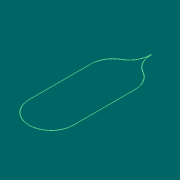
# Autodesk Inventor part: Fiber Loop
Saved by Autodesk Inventor 2016 (Build 200138000, 138)
## iProperties
Created: 2015-08-17
Part Number: Fiber Loop
Material: Glass
Document SubType Name: Modeling
Designer: Cosmic
Density: 2.18 g/cm^3
Appearance: Clear - Green 1
Author: Cosmic
Autodesk Inventor part; units mm, degrees
ref_plane "YZ Plane" through (0, 0, 0) normal (1, 0, 0) x (0, 1, 0)
ref_plane "XZ Plane" through (0, 0, 0) normal (0, 1, 0) x (-1, 0, 0)
ref_plane "XY Plane" through (0, 0, 0) normal (0, 0, 1) x (1, 0, 0)
sketch "Sketch1" plane through (0, 0, 0) normal (0, 0, 1) x (1, 0, 0)
  arc A0 (1.300022, 83.780057) -> (24.510414, 44.495838) centre (46.150022, 83.780057) ccw
  line L0 (-49.5, 0) -> (-49.5, -140)
  line L1 (49.5, 0) -> (49.5, -140)
  line L2 (0, 0) -> (0, -140)
  line L3 (-1.300022, 83.780057) -> (1.300022, 83.780057)
  arc A1 (49.5, 0) -> (23.883179, 43.357165) centre (0, 0) ccw
  arc A2 (-49.5, -140) -> (49.5, -140) centre (0, -140) ccw
  line L4 (-50.8, -140) -> (-50.8, 0)
  arc A3 (50.8, 0) -> (49.5, 11.418844) centre (0, 0) ccw
  line L5 (50.8, 0) -> (50.8, -140)
  arc A4 (-50.8, -140) -> (50.8, -140) centre (0, -140) ccw
  arc A5 (-17.703412, 47.455377) -> (-17.32803, 47.75333) centre (-46.299935, 83.868683) ccw
  line L6 (0, 83.780057) -> (0, 0)
  line L7 (-50.65, 0) -> (-50.65, -140)
  arc A6 (-50.65, -140) -> (50.65, -140) centre (0, -140) ccw
  line L8 (50.65, -140) -> (50.65, 0)
  arc A7 (50.65, 0) -> (49.5, 10.731845) centre (0, 0) ccw
  line L9 (-49.65, 0) -> (-49.65, -140)
  arc A8 (-49.65, -140) -> (49.65, -140) centre (0, -140) ccw
  line L10 (49.65, -140) -> (49.65, 0)
  arc A9 (49.65, 0) -> (49.5, 3.856488) centre (0, 0) ccw
  arc A10 (-18.180609, 47.274612) -> (-17.777737, 47.587742) centre (-46.299935, 83.868683) ccw
  arc A11 (-24.479037, 44.341846) -> (-22.173914, 45.70512) centre (-46.299935, 83.868683) ccw
  arc A12 (-23.923244, 43.335071) -> (-49.5, 0) centre (0, 0) ccw
  arc A13 (-26.306888, 42.107839) -> (-49.5, 3.856488) centre (0, 0) ccw
  arc A14 (-23.995739, 43.46639) -> (-26.306888, 42.107839) centre (0, 0) ccw
  arc A15 (-23.995739, 43.46639) -> (-18.180609, 47.274612) centre (-46.299935, 83.868683) ccw
  arc A16 (-21.614599, 44.698233) -> (-17.703412, 47.455377) centre (-46.299935, 83.868683) ccw
  arc A17 (-24.479037, 44.341846) -> (-30.316871, 40.574744) centre (0, 0) ccw
  arc A18 (-24.551531, 44.473164) -> (-1.300022, 83.780057) centre (-46.299935, 83.868683) ccw
  arc A19 (-24.551531, 44.473164) -> (-26.860934, 43.117632) centre (0, 0) ccw
  arc A20 (-30.316871, 40.574744) -> (-50.65, 0) centre (0, 0) ccw
  arc A21 (-26.860934, 43.117632) -> (-30.796483, 40.400701) centre (0, 0) ccw
  arc A22 (-30.796483, 40.400701) -> (-50.8, 0) centre (0, 0) ccw
  arc A23 (-49.5, 3.856488) -> (-49.65, 0) centre (0, 0) ccw
  arc A24 (-23.923244, 43.335071) -> (-21.614599, 44.698233) centre (-46.299935, 83.868683) ccw
  arc A25 (-17.777737, 47.587742) -> (-0.15002, 83.780057) centre (-46.299935, 83.868683) ccw
  arc A26 (-22.173914, 45.70512) -> (-1.150022, 83.780057) centre (-46.299935, 83.868683) ccw
  arc A27 (26.306921, 42.107819) -> (23.955553, 43.48855) centre (0, 0) ccw
  arc A28 (26.819027, 43.143711) -> (24.510414, 44.495838) centre (0, 0) ccw
  arc A29 (30.753984, 40.433062) -> (26.819027, 43.143711) centre (0, 0) ccw
  arc A30 (22.104154, 45.743283) -> (24.438041, 44.364452) centre (46.150022, 83.780057) ccw
  arc A31 (1.150022, 83.780057) -> (22.104154, 45.743283) centre (46.150022, 83.780057) ccw
  arc A32 (17.290361, 47.76697) -> (17.646145, 47.48472) centre (46.150022, 83.780057) ccw
  arc A33 (17.646145, 47.48472) -> (21.544661, 44.736508) centre (46.150022, 83.780057) ccw
  arc A34 (21.544661, 44.736508) -> (23.883179, 43.357165) centre (46.150022, 83.780057) ccw
  arc A35 (18.122092, 47.304927) -> (23.955553, 43.48855) centre (46.150022, 83.780057) ccw
  arc A36 (49.5, 3.856488) -> (26.306921, 42.107819) centre (0, 0) ccw
  arc A37 (30.316871, 40.574744) -> (24.438041, 44.364452) centre (0, 0) ccw
  arc A38 (0.000044, 83.824298) -> (17.290361, 47.76697) centre (46.150022, 83.780057) ccw
  arc A39 (17.720529, 47.617039) -> (18.122092, 47.304927) centre (46.150022, 83.780057) ccw
  arc A40 (0.150022, 83.780057) -> (17.720529, 47.617039) centre (46.150022, 83.780057) ccw
  arc A41 (31.176261, 40.108363) -> (30.753984, 40.433062) centre (0, 0) ccw
  arc A42 (49.5, 11.418844) -> (31.176261, 40.108363) centre (0, 0) ccw
  arc A43 (30.724109, 40.267253) -> (30.316871, 40.574744) centre (0, 0) ccw
  arc A44 (49.5, 10.731845) -> (30.724109, 40.267253) centre (0, 0) ccw
  arc A45 (-17.32803, 47.75333) -> (0.000044, 83.824298) centre (-46.299935, 83.868683) ccw
  dimension "d44" = 140
  dimension "d45" = 49.5
  dimension "d48" = 1.3
  dimension "d49" = 0.15
  dimension "d50" = 0.15
  dimension "d53" = 0.15
  dimension "d55" = 0.15
  dimension "d56" = 0.15
  dimension "d57" = 1.3
  dimension "d58" = 1.3
  dimension "d61" = 45
  dimension "d62" = 1.3
  dimension "d63" = 1.3
  dimension "d64" = 1.3
  dimension "d65" = 0.15
  dimension "d66" = 0.15
  dimension "d67" = 45
  constraints: 107 point on circle, 46 centre point, 22 end point, 12 tangent, 9 point on line, 4 parallel, 2 midpoint, 1 coincident, 1 horizontal, 1 line through centre, 1 perpendicular, 1 vertical, 6 other
  measures "d44" distance of L2.start L2.end
  measures "d45" radius of A1
  measures "d48" radial gap between concentric circles of A3 A1
  measures "d49" radial gap between concentric circles of A3 A7
  measures "d50" radial gap between concentric circles of A1 A9
  measures "d53" radial gap between concentric circles of A10 A5
  measures "d55" distance between parallel lines of L10 L1
  measures "d56" distance between parallel lines of L5 L8
  measures "d57" distance between parallel lines of L1 L5
  measures "d58" distance between parallel lines of L0 L4
  measures "d61" radius of A18
  measures "d62" radial gap between concentric circles of A22 A12
  measures "d63" radial gap between concentric circles of A0 A38
  measures "d64" radial gap between concentric circles of A18 A45
  measures "d65" radial gap between concentric circles of A22 A20
  measures "d66" radial gap between concentric circles of A12 A23
  measures "d67" radius of A31
sketch "Sketch1 outline for Extrusion3" plane through (0, 0, 0) normal (0, 0, 1) x (1, 0, 0)
  arc A0 (-30.316871, 40.574744) -> (-50.65, 0) centre (0, 0) ccw
  arc A1 (-24.479037, 44.341846) -> (-30.316871, 40.574744) centre (0, 0) ccw
  arc A2 (-22.173914, 45.70512) -> (-24.479037, 44.341846) centre (-46.299935, 83.868683) cw
  arc A3 (-1.150022, 83.780057) -> (-22.173914, 45.70512) centre (-46.299935, 83.868683) cw
  line L0 (-0.15002, 83.780057) -> (-1.150022, 83.780057)
  arc A4 (-17.777737, 47.587742) -> (-0.15002, 83.780057) centre (-46.299935, 83.868683) ccw
  arc A5 (-18.180609, 47.274612) -> (-17.777737, 47.587742) centre (-46.299935, 83.868683) ccw
  arc A6 (-23.995739, 43.46639) -> (-18.180609, 47.274612) centre (-46.299935, 83.868683) ccw
  arc A7 (-26.306888, 42.107839) -> (-23.995739, 43.46639) centre (0, 0) cw
  arc A8 (-49.5, 3.856488) -> (-26.306888, 42.107839) centre (0, 0) cw
  arc A9 (-49.65, 0) -> (-49.5, 3.856488) centre (0, 0) cw
  line L1 (-49.65, -140) -> (-49.65, 0)
  arc A10 (49.65, -140) -> (-49.65, -140) centre (0, -140) cw
  line L2 (49.65, 0) -> (49.65, -140)
  arc A11 (49.5, 3.856488) -> (49.65, 0) centre (0, 0) cw
  arc A12 (26.306921, 42.107819) -> (49.5, 3.856488) centre (0, 0) cw
  arc A13 (23.955553, 43.48855) -> (26.306921, 42.107819) centre (0, 0) cw
  arc A14 (18.122092, 47.304927) -> (23.955553, 43.48855) centre (46.150022, 83.780057) ccw
  arc A15 (17.720529, 47.617039) -> (18.122092, 47.304927) centre (46.150022, 83.780057) ccw
  arc A16 (0.150022, 83.780057) -> (17.720529, 47.617039) centre (46.150022, 83.780057) ccw
  line L3 (1.150022, 83.780057) -> (0.150022, 83.780057)
  arc A17 (22.104154, 45.743283) -> (1.150022, 83.780057) centre (46.150022, 83.780057) cw
  arc A18 (24.438041, 44.364452) -> (22.104154, 45.743283) centre (46.150022, 83.780057) cw
  arc A19 (30.316871, 40.574744) -> (24.438041, 44.364452) centre (0, 0) ccw
  arc A20 (30.724109, 40.267253) -> (30.316871, 40.574744) centre (0, 0) ccw
  arc A21 (49.5, 10.731845) -> (30.724109, 40.267253) centre (0, 0) ccw
  arc A22 (50.65, 0) -> (49.5, 10.731845) centre (0, 0) ccw
  line L4 (50.65, -140) -> (50.65, 0)
  arc A23 (-50.65, -140) -> (50.65, -140) centre (0, -140) ccw
  line L5 (-50.65, 0) -> (-50.65, -140)
extrude "Extrusion3" add sketch "Sketch1 outline for Extrusion3" along normal blind 1
sketch "Sketch3" plane through (-1.150022, 83.780057, 0) normal (0, 1, 0) x (1, 0, 0)
  line L0 (2.300045, 0) -> (1.300045, 0)
  line L1 (1.300045, 0) -> (1.300045, -1)
  line L2 (2.300045, -1) -> (1.300045, -1)
  line L3 (2.300045, 0) -> (2.300045, -1)
  line L4 (1.000002, 0) -> (0, 0)
  line L5 (0, 0) -> (0, -1)
  line L6 (1.000002, -1) -> (0, -1)
  line L7 (1.000002, 0) -> (1.000002, -1)
  point P0 (1.150022, 0)
extrude "Extrusion4" add sketch "Sketch3" along normal blind 3
fillet "Fillet2" radius 0.495 36 edges at (6.5461, 60.3808, 0) (42.7464, 25.256, 0) (49.65, -70, 0) (0, -189.65, 0) (-49.65, -70, 0) (-42.7581, 25.2362, 0) (-6.5785, 60.3733, 0) (0.15, 85.2801, 0) (-0.15, 85.2801, 0) (49.65, -70, 1) (0, -189.65, 1) (-49.65, -70, 1) (-42.7581, 25.2362, 1) (-6.5785, 60.3733, 1) (6.5461, 60.3808, 1) (0.15, 85.2801, 1) (42.7464, 25.256, 1) (-0.15, 85.2801, 1) (7.407, 60.8894, 0) (43.6074, 25.7647, 0) (50.65, -70, 0) (0, -190.65, 0) (-50.65, -70, 0) (-43.6193, 25.7445, 0) (-7.4397, 60.8816, 0) (1.15, 85.2801, 0) (7.407, 60.8894, 1) (43.6074, 25.7647, 1) (50.65, -70, 1) (0, -190.65, 1) (-50.65, -70, 1) (-43.6193, 25.7445, 1) (-7.4397, 60.8816, 1) (1.15, 85.2801, 1) (-1.15, 85.2801, 1) (-1.15, 85.2801, 0)
equation "\"d44\" = LoopLength"
equation "\"d48\" = OpticalFiberDiameter + 2 * OpticalFiberClearence"
equation "\"d49\" = OpticalFiberClearence"
equation "\"d50\" = OpticalFiberClearence"
equation "\"d53\" = OpticalFiberClearence"
equation "\"d55\" = OpticalFiberClearence"
equation "\"d56\" = OpticalFiberClearence"
equation "\"d57\" = OpticalFiberDiameter + 2 * OpticalFiberClearence"
equation "\"d58\" = OpticalFiberDiameter + 2 * OpticalFiberClearence"
equation "\"d61\" = 0.5 * LoopSmallTrackDiameter"
equation "\"d59\" = OpticalFiberDiameter"
equation "\"OpticalFiberDiameter\" = 1"
equation "\"OpticalFiberClearence\" = 0.15"
equation "\"ScintillatorEdgeClearence\" = 3"
equation "\"MPPCDepth\" = 1"
equation "\"LoopLargeTrackRatio\" = 1.1"
equation "\"d24\" = 0.05"
equation "\"d25\" = 1"
equation "\"d32\" = 0.05"
equation "\"d33\" = 1"
equation "\"FiberSensorClerence\" = 0.5"
equation "\"SmallTrackDiameter\" = 175"
equation "\"ScintillatorWidth\" = 145"
equation "\"ShallowTrackDepth\" = 1.3"
equation "\"MPPCClearence\" = 0.075"
equation "\"MPPCSensorClearence\" = 1.45"
equation "\"MPPCSensorOffsett\" = 2.105"
equation "\"MPPCWidth\" = 5.9"
equation "\"MPPCHeight\" = 6.55"
equation "\"FiberEdgeOffsett\" = 5"
equation "\"LongFiberAngle\" = 30deg"
equation "\"ShortFiberAngle\" = 78deg"
equation "\"MountingScrewOffsett\" = 12"
equation "\"MountingScrewDepth\" = 5"
equation "\"LoopLength\" = 140"
equation "\"d46\" = OpticalFiberDiameter + 2 * OpticalFiberClearence"
equation "\"d54\" = OpticalFiberClearence"
equation "\"LoopSmallTrackDiameter\" = 90"
body "Solid1"
body "Solid2"
